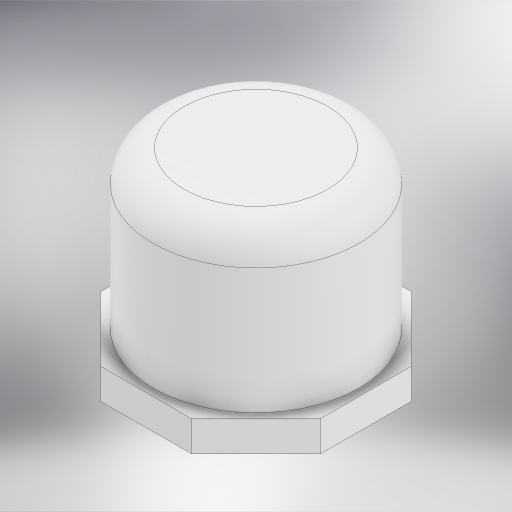
# Autodesk Inventor part: Tapón
Saved by Autodesk Inventor 2023 (Build 270158000, 158)
## iProperties
Created: 2023-02-27
Part Number: Tapón
Material: PVC, no plastificado
Document SubType Name: Modeling
Designer: Braya
Density: 1.29 g/cm^3
Appearance: Suave - Blanco
Mass: 15.5237 g
Surface Area: 70.8612 cm^2
Volume: 12.0339 cm^3
Author: Braya
Autodesk Inventor part; units mm, degrees
ref_plane "YZ Plane" through (0, 0, 0) normal (1, 0, 0) x (0, 1, 0)
ref_plane "XZ Plane" through (0, 0, 0) normal (0, 1, 0) x (-1, 0, 0)
ref_plane "XY Plane" through (0, 0, 0) normal (0, 0, 1) x (1, 0, 0)
sketch "Boceto1" plane through (0, 0, 0) normal (0, 1, 0) x (-1, 0, 0)
  circle A0 centre (0, 0) radius 16.5
  dimension "d0" = 33
  constraints: 1 centre point, 1 coincident
  measures "d0" diameter of A0
extrude "Extrusión1" add sketch "Boceto1" along normal blind 30
sketch "Boceto2" plane through (0, 0, 0) normal (0, -1, 0) x (1, 0, 0)
  line L0 (-7.2902, 17.6) -> (7.2902, 17.6)
  line L1 (17.6, 7.2902) -> (17.6, -7.2902)
  line L2 (7.2902, -17.6) -> (-7.2902, -17.6)
  line L3 (-17.6, -7.2902) -> (-17.6, 7.2902)
  line L4 (-17.6, 17.6) -> (17.6, -17.6) construction
  line L5 (17.6, 17.6) -> (-17.6, -17.6) construction
  line L6 (-17.6, 7.2902) -> (-7.2902, 17.6)
  line L7 (-24.8902, 0) -> (10.3098, 0) construction
  line L8 (7.2902, 17.6) -> (17.6, 7.2902)
  line L9 (17.6, -7.2902) -> (7.2902, -17.6)
  line L10 (-7.2902, -17.6) -> (-17.6, -7.2902)
  line L11 (-24.8902, 0) -> (24.8902, 0)
  line L12 (0, -24.8902) -> (0, 24.8902)
  point P0 (0, 0)
  point P1 (0, 0)
  dimension "d3" = 35.2
  dimension "d4" = 35.2
  dimension "d5" = 35.2
  dimension "d6" = 45
  dimension "d7" = 35.2
  constraints: 26 end point, 4 midpoint, 4 perpendicular, 2 horizontal, 2 parallel
  measures "d3" distance of L4.end L5.end
  measures "d4" distance of L5.start L4.end
  measures "d5" distance of L7.start L12.end
  measures "d6" angle of L7 L6
  measures "d7" distance of L12.end L11.end
extrude "Extrusión2" add sketch "Boceto2" against normal blind 4.9
fillet "Empalme1" radius 5 1 edges at (16.5, 30, 0)
sketch "Boceto3" plane through (0, 0, 0) normal (0, -1, 0) x (1, 0, 0)
  circle A0 centre (0, 0) radius 13.325
  dimension "d11" = 26.65
  constraints: 1 centre point, 1 coincident
  measures "d11" diameter of A0
extrude "Extrusión3" cut sketch "Boceto3" against normal blind 25
